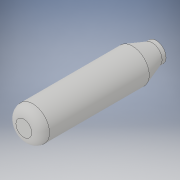
# Autodesk Inventor part: volume_reservoir
Saved by Autodesk Inventor 2019 (Build 230136000, 136)
## iProperties
Created: 2018-04-28
Part Number: volume_reservoir
Material: Générique
Document SubType Name: Modeling
Designer: Theo
Mass: 111.198 g
Surface Area: 145.717 cm^2
Volume: 111.198 cm^3
Density: 1 g/cm^3
Appearance: Par défaut
Author: Theo
Autodesk Inventor part; units mm, degrees
ref_plane "YZ Plane" through (0, 0, 0) normal (1, 0, 0) x (0, 1, 0)
ref_plane "XZ Plane" through (0, 0, 0) normal (0, 1, 0) x (-1, 0, 0)
ref_plane "XY Plane" through (0, 0, 0) normal (0, 0, 1) x (1, 0, 0)
sketch "Esquisse1" plane through (0, 0, 0) normal (1, 0, 0) x (0, 1, 0)
  line L0 (0, 9.746) -> (0, -11.8589)
  line L1 (17, -9) -> (17, -110)
  arc A0 (17, -9) -> (8, 0) centre (8, -9) ccw
  line L2 (17, -110) -> (10, -130)
  line L3 (10, -130) -> (10, -134)
  line L4 (8, 0) -> (0, 0)
  line L5 (0, 0) -> (0, -134)
  line L6 (0, -134) -> (10, -134)
  dimension "d0" = 34
  dimension "d1" = 20
  dimension "d2" = 4
  dimension "d3" = 20
  dimension "d4" = 9
  dimension "d5" = 130
  constraints: 14 end point, 4 vertical, 2 horizontal, 2 point on circle, 2 tangent, 1 centre point, 1 point on line
  measures "d0" diameter of L1 L0
  measures "d1" vertical distance of L1.end L2.end
  measures "d2" distance of L2.end L3.end
  measures "d3" diameter of L2.end L0
  measures "d4" radius of A0
  measures "d5" vertical distance of L2.end L4.end
revolve "Révolution1" add sketch "Esquisse1" angle 360 about axis through (0, 0, 9.746) along (0, 0, -1)
